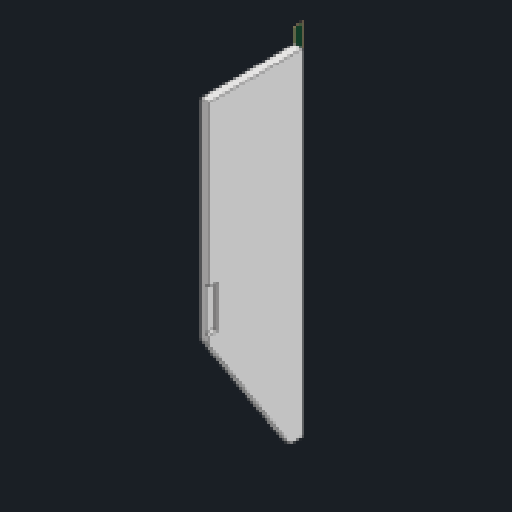
# Autodesk Inventor part: right_side
Saved by Autodesk Inventor 2023 (Build 270158000, 158)
## iProperties
Created: 2024-04-23
Part Number: right_side
Material: Generic
Document SubType Name: Modeling
Designer: szymo
Density: 1 g/cm^3
Appearance: Default
Author: szymo
Autodesk Inventor part; units mm, degrees
ref_plane "YZ Plane" through (0, 0, 0) normal (1, 0, 0) x (0, 1, 0)
ref_plane "XZ Plane" through (0, 0, 0) normal (0, 1, 0) x (-1, 0, 0)
ref_plane "XY Plane" through (0, 0, 0) normal (0, 0, 1) x (1, 0, 0)
ref_plane "Work Plane4" through (-12.2663, 34.5, -3) normal (-1, 0, 0) x (0, 0, 1)
sketch "Sketch4" plane through (-12.2663, 34.5, -3) normal (-1, 0, 0) x (0, 0, 1)
  line L0 (0, 0) -> (0, -108) projected
  line L1 (0, -108) -> (3, -108) projected
  line L2 (3, 0) -> (3, -108) projected
  line L3 (0, 0) -> (3, 0) projected
  circle A0 centre (13.5, 27.5) radius 25 projected
  line L4 (7.5, -120) -> (3, -120) projected
  line L5 (3, -120) -> (3, -124) projected
  line L6 (3, -124) -> (-0.5, -124) projected
  line L7 (-0.5, -124) -> (-0.5, -138) projected
  line L8 (-0.5, -138) -> (8.5, -124) projected
  line L9 (8.5, -124) -> (7.5, -124) projected
  line L10 (7.5, -124) -> (7.5, -120) projected
  line L11 (0, -111) -> (3, -111) projected
  line L12 (0, -111) -> (0, -124) projected
  line L13 (0, -124) -> (3, -124) projected
  line L14 (3, -111) -> (3, -124) projected
  line L15 (3, -111) -> (3, -108) projected
  line L16 (0, -108) -> (0, -111) projected
  line L17 (7.5, -120) -> (3, -120)
  line L18 (3, -120) -> (3, 0)
  line L19 (3, 0) -> (36.5, 0)
  line L20 (8.5, -124) -> (66.1149, -34.3768)
  line L21 (7.5, -120) -> (63.7229, -32.5421)
  line L22 (36.5, 0) -> (36.5, -74.8889)
  line L23 (36.5, -72.0889) -> (33.5, -72.0889)
  line L24 (33.5, -72.0889) -> (33.5, -56.9889)
  line L25 (33.5, -56.9889) -> (36.5, -56.9889)
  line L26 (36.5, -56.9889) -> (36.5, -72.0889)
  point P0 (3, -34.5)
  point P1 (38.5, 27.5)
  point P2 (36.5, -56.9889)
  dimension "d4" = 25
  dimension "d5" = 2
  dimension "d9" = 2.8
  dimension "d10" = 15.1
  dimension "d11" = 3
  constraints: 20 end point, 3 horizontal, 3 parallel, 2 collinear, 2 point on line, 1 horizontal alignment, 1 perpendicular, 1 vertical, 1 other
  measures "d4" distance of point (13.5, 27.5) point (38.5, 27.5)
  measures "d5" distance from line of point (38.5, 27.5) L22
  measures "d9" distance from line of L23 L22.end
  measures "d10" distance of L23.end L24.end
  measures "d11" distance between parallel lines of L26 L24
extrude "Extrusion1" add sketch "Sketch4" against normal blind 3 contours L19 L22 L25 L24 L23 L21 L4 L14 L15 L2
sketch "Sketch8" plane through (-12.2663, -37.5889, 30.5) normal (0, 0, 1) x (1, 0, 0)
  line L0 (22.5, 14.9) -> (2, 14.9) projected
  line L1 (1.9, 14.8) -> (1.9, 0.3) projected
  line L2 (2, 0.2) -> (22.5, 0.2) projected
  line L3 (0, 0) -> (0, 15.1) projected
  line L4 (0, 0) -> (3, 0) projected
  line L5 (3, 15.1) -> (3, 0) projected
  line L6 (0, 15.1) -> (3, 15.1) projected
  line L7 (0, -2.8) -> (0, 0) projected
  line L8 (0, -2.8) -> (3, -2.8) projected
  line L9 (3, 0) -> (3, -2.8) projected
  line L10 (0, 0) -> (3, 0) projected
  line L11 (0, 15.1) -> (0, 72.0889) projected
  line L12 (0, 15.1) -> (3, 15.1) projected
  line L13 (3, 72.0889) -> (3, 15.1) projected
  line L14 (0, 72.0889) -> (3, 72.0889) projected
  line L15 (0, 15.1) -> (1.7, 15.1)
  line L16 (1.7, 15.1) -> (1.7, 0)
  line L17 (1.7, 0) -> (0, 0)
  line L18 (0, 0) -> (0, 15.1)
  point P0 (12.2663, 37.5889)
  point P1 (1.7, 0)
  point P2 (1.7, 15.1)
  dimension "d12" = 0.2
  constraints: 8 end point, 2 parallel, 1 horizontal, 1 perpendicular, 1 point on line
  measures "d12" distance between parallel lines of L16 L1
extrude "Extrusion2" add sketch "Sketch8" along normal up to surface (3 mm away) contours L3 L6 L16 L4
body "Solid1"
